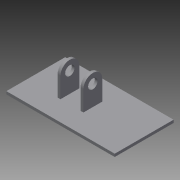
# Autodesk Inventor part: Foot
Saved by Autodesk Inventor 2013 (Build 170138000, 138)
## iProperties
Created: 2012-11-29
Part Number: Foot
Material: Generic
Document SubType Name: Modeling
Designer: Joe
Density: 1 g/cm^3
Author: Joe
Autodesk Inventor part; units mm, degrees
ref_plane "YZ Plane" through (0, 0, 0) normal (1, 0, 0) x (0, 1, 0)
ref_plane "XZ Plane" through (0, 0, 0) normal (0, 1, 0) x (-1, 0, 0)
ref_plane "XY Plane" through (0, 0, 0) normal (0, 0, 1) x (1, 0, 0)
sketch "Sketch2" plane through (0, 0, 0) normal (1, 0, 0) x (0, 1, 0)
  line L0 (20, 27.3876) -> (-42.6897, 27.3876)
  line L1 (-42.6897, 21.3876) -> (20, 21.3876)
  line L2 (20, 21.3876) -> (20, 27.3876)
  line L3 (-42.6897, -21.3876) -> (20, -21.3876)
  line L4 (20, -21.3876) -> (20, -27.3876)
  line L5 (20, -27.3876) -> (-42.6897, -27.3876)
  line L6 (-42.6897, -93.6124) -> (-48.6897, -93.6124)
  line L7 (-48.6897, -93.6124) -> (-48.6897, 136.3876)
  line L8 (-48.6897, 136.3876) -> (-42.6897, 136.3876)
  line L9 (-42.6897, 136.3876) -> (-42.6897, 27.3876)
  line L10 (-42.6897, 21.3876) -> (-42.6897, -21.3876)
  line L11 (-42.6897, -27.3876) -> (-42.6897, -93.6124)
  point P0 (0, 0)
  dimension "d3" = 6
  dimension "d5" = 48.6897
  dimension "d6" = 136.3876
  dimension "d7" = 93.6124
  dimension "d9" = 27.3876
  dimension "d10" = 27.3876
  dimension "d11" = 20
  constraints: 24 end point, 6 parallel, 3 collinear, 3 horizontal, 2 equal length, 2 perpendicular
  measures "d3" distance of L3.end L4.end
  measures "d5" distance from line of L7 point (0, 0)
  measures "d6" distance from line of L8 point (0, 0)
  measures "d7" distance from line of L6 point (0, 0)
  measures "d9" distance from line of L5 point (0, 0)
  measures "d10" distance from line of point (0, 0) L0
  measures "d11" distance from line of L2 point (0, 0)
extrude "Extrusion1" add sketch "Sketch2" along normal mid plane 125
sketch "Sketch3" plane through (-62.5, -42.6897, 27.3876) normal (0, 0, 1) x (1, 0, 0)
  circle A0 centre (62.5, 42.6897) radius 10
  dimension "d14" = 20
  constraints: 1 centre point, 1 coincident
  measures "d14" diameter of A0
extrude "Extrusion2" cut sketch "Sketch3" against normal through all
sketch "Sketch4" plane through (-62.5, -42.6897, 27.3876) normal (0, 0, 1) x (1, 0, 0)
  circle A0 centre (62.5, 42.6897) radius 10 projected
  line L0 (0, 0) -> (125, 0) projected
  line L1 (125, 62.6897) -> (125, 0) projected
  line L2 (125, 62.6897) -> (0, 62.6897) projected
  line L3 (0, 0) -> (0, 62.6897) projected
  arc A1 (82.5, 42.6897) -> (42.5, 42.6897) centre (62.5, 42.6897) ccw
  line L4 (42.5, 42.6897) -> (42.5, 0)
  line L5 (82.5, 0) -> (82.5, 42.6897)
  constraints: 4 end point, 2 point on circle, 2 point on line, 2 tangent, 1 centre point, 1 coincident, 1 perpendicular
extrude "Extrusion3" cut sketch "Sketch4" against normal through all contours L3 L2 A1 L4 L0 | L5 A1 L2 L1 L0
move or copy body "Move Body1" bodies to move or copy 1 copy no rotation origin (0, 0, 0) rotation axis (1, 0, 0) rotation angle 90
move or copy body "Move Body2" bodies to move or copy 1 copy no rotation origin (0, 0, 0) rotation axis (0, 0, 1) rotation angle 90
body "Solid1"
